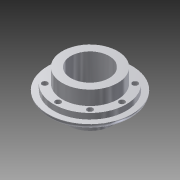
# Autodesk Inventor part: X-Ray Tube Output
Saved by Autodesk Inventor 2015 (Build 190159000, 159)
## iProperties
Created: 2015-03-09
Part Number: X-Ray Tube Output
Material: Aluminum 6061
Document SubType Name: Modeling
Designer: pltwe4
Density: 2.7 g/cm^3
Appearance: Aluminum - Flat
Author: pltwe4
Autodesk Inventor part; units mm, degrees
ref_plane "YZ Plane" through (0, 0, 0) normal (1, 0, 0) x (0, 1, 0)
ref_plane "XZ Plane" through (0, 0, 0) normal (0, 1, 0) x (-1, 0, 0)
ref_plane "XY Plane" through (0, 0, 0) normal (0, 0, 1) x (1, 0, 0)
sketch "Sketch1" plane through (0, 0, 0) normal (0, 0, 1) x (1, 0, 0)
  circle A0 centre (0, 0) radius 7.75
  circle A1 centre (0, 0) radius 9.75
  circle A2 centre (0, 0) radius 6.75
  circle A3 centre (0, 0) radius 14.75
  dimension "d0" = 15.5
  dimension "d1" = 2
  dimension "d2" = 1
  dimension "d5" = 5
  constraints: 4 centre point, 2 coincident
  measures "d0" diameter of A0
  measures "d1" radial gap between concentric circles of A0 A1
  measures "d2" radial gap between concentric circles of A2 A0
  measures "d5" radial gap between concentric circles of A3 A1
extrude "Extrusion1" add sketch "Sketch1" against normal blind 5 contours A0
extrude "Extrusion2" add sketch "Sketch1" along normal blind 2 contours A0 | A1 | A3
fillet "Fillet1" radius 2 1 edges at (-14.75, 0, 0)
sketch "Sketch2" plane through (0, 0, 2) normal (0, 0, 1) x (1, 0, 0)
  circle A0 centre (0, 0) radius 12.75
  circle A1 centre (0, 0) radius 6.75
  dimension "d9" = 25.5
  dimension "d10" = 13.5
  constraints: 2 centre point, 2 coincident
  measures "d9" diameter of A0
  measures "d10" diameter of A1
extrude "Extrusion3" add sketch "Sketch2" along normal blind 2
sketch "Sketch3" plane through (0, 0, 4) normal (0, 0, 1) x (1, 0, 0)
  circle A0 centre (0, 0) radius 6.75 projected
  circle A1 centre (0, 0) radius 9.75
  dimension "d13" = 3
  constraints: 1 centre point, 1 coincident
  measures "d13" radial gap between concentric circles of A0 A1
extrude "Extrusion4" add sketch "Sketch3" along normal blind 5
sketch "Sketch4" plane through (0, 0, 4) normal (0, 0, 1) x (1, 0, 0)
  circle A0 centre (0, 0) radius 9.75 projected
  circle A1 centre (0, 0) radius 12.75 projected
  line L0 (0, 20.65) -> (0, -20.65) construction
  circle A2 centre (0, 0) radius 9.75 construction
  line L1 (0, 9.75) -> (0, 12.75) construction
  line L2 (0, 11.25) -> (0.6069, 11.25) construction
  dimension "d27" = 25.5
  constraints: 4 end point, 2 point on line, 2 vertical alignment, 1 coincident, 1 horizontal, 1 midpoint, 2 other
hole "Hole1" at (0, 11.25, 4) direction (0, 0, -1) diameter 2 depth 3 tip angle 118
pattern_circular "Circular Pattern1" count 8 over 360 about axis through (0, 0, 0) along (0, 0, -1) of "Hole1"
body "Solid1"
